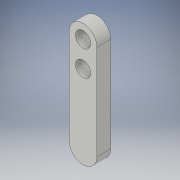
# Autodesk Inventor part: Brake
Saved by Autodesk Inventor 2018 (Build 220112000, 112)
## iProperties
Created: 2019-07-16
Part Number: Brake
Material: Generic
Document SubType Name: Modeling
Designer: anirudh
Density: 1 g/cm^3
Appearance: Default
Author: anirudh
Autodesk Inventor part; units mm, degrees
ref_plane "YZ Plane" through (0, 0, 0) normal (1, 0, 0) x (0, 1, 0)
ref_plane "XZ Plane" through (0, 0, 0) normal (0, 1, 0) x (-1, 0, 0)
ref_plane "XY Plane" through (0, 0, 0) normal (0, 0, 1) x (1, 0, 0)
sketch "Sketch1" plane through (0, 0, 0) normal (0, 0, 1) x (1, 0, 0)
  circle A0 centre (0, 0) radius 1.75
  circle A1 centre (0, -5.8674) radius 1.75
  arc A2 (-3.175, -15.3924) -> (3.175, -15.3924) centre (0, -15.3924) ccw
  arc A3 (3.175, 0) -> (-3.175, 0) centre (0, 0) ccw
  line L0 (-3.175, 0) -> (-3.175, -15.3924)
  line L1 (3.175, 0) -> (3.175, -15.3924)
  dimension "d0" = 3.5
  dimension "d3" = 3.5
  constraints: 4 centre point, 4 end point, 4 point on circle, 2 coincident, 2 vertical
  measures "d0" diameter of A0
  measures "d3" diameter of A1
extrude "Extrusion1" add sketch "Sketch1" along normal blind 3.175
sketch "Sketch2" plane through (0, 0, 3.175) normal (0, 0, 1) x (1, 0, 0)
  arc A0 (-3.175, -15.3924) -> (3.175, -15.3924) centre (0, -15.3924) ccw projected
  arc A1 (-3.175, -21.7424) -> (3.175, -21.7424) centre (0, -21.7424) ccw
  line L0 (-3.175, 0) -> (-3.175, -15.3924) projected
  line L1 (-3.175, -21.7424) -> (-3.175, -15.3924)
  line L2 (3.175, -15.3924) -> (3.175, -21.7424)
  arc A2 (-3.175, -15.3924) -> (3.175, -15.3924) centre (0, -15.3924) ccw
  point P0 (0, 0)
  dimension "d10" = 6.35
  constraints: 4 end point, 4 point on circle, 2 centre point, 2 vertical, 1 coincident
  measures "d10" diameter of A1
extrude "Extrusion2" add sketch "Sketch2" against normal blind 3.175
body "Solid1"
